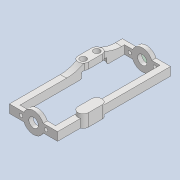
# Autodesk Inventor part: cable_holder_1
Saved by Autodesk Inventor 2020 (Build 240168000, 168)
## iProperties
Created: 2021-07-19
Part Number: cable_holder_1
Material: Generic
Document SubType Name: Modeling
Designer: Shuang Peng
Density: 1 g/cm^3
Appearance: Default
Author: Shuang Peng
Autodesk Inventor part; units mm, degrees
ref_plane "YZ Plane" through (0, 0, 0) normal (1, 0, 0) x (0, 1, 0)
ref_plane "XZ Plane" through (0, 0, 0) normal (0, 1, 0) x (-1, 0, 0)
ref_plane "XY Plane" through (0, 0, 0) normal (0, 0, 1) x (1, 0, 0)
sketch "Sketch1" plane through (0, 0, 0) normal (0, 0, 1) x (1, 0, 0)
  circle A0 centre (0, 0) radius 5
  line L0 (-15, 2) -> (-15, -2)
  line L1 (-15, -2) -> (15, -2)
  line L2 (15, -2) -> (15, 2)
  line L3 (15, 2) -> (-15, 2)
  line L4 (-15, 2) -> (15, -2) construction
  line L5 (-15, -2) -> (15, 2) construction
  point P0 (4.5826, 2)
  point P1 (-4.5826, 2)
  point P2 (-4.5826, -2)
  point P3 (4.5826, -2)
  dimension "d0" = 10
  dimension "d1" = 4
  dimension "d2" = 30
  constraints: 12 end point, 2 midpoint, 2 parallel, 1 centre point, 1 coincident, 1 perpendicular, 1 vertical
  measures "d0" diameter of A0
  measures "d1" distance of L0.start L0.end
  measures "d2" distance of L1.end L0.end
extrude "Extrusion1" add sketch "Sketch1" against normal blind 2
ref_plane "Work Plane1" through (0, 0, -54) normal (0, 0, -1) x (1, 0, 0)
sketch "Sketch2" plane through (0, 0, -54) normal (0, 0, -1) x (1, 0, 0)
  circle A0 centre (0, 0) radius 5
  line L0 (15, 2) -> (15, -2)
  line L1 (15, -2) -> (-15, -2)
  line L2 (-15, -2) -> (-15, 2)
  line L3 (-15, 2) -> (15, 2)
  line L4 (15, 2) -> (-15, -2) construction
  line L5 (15, -2) -> (-15, 2) construction
  point P0 (-4.5826, 2)
  point P1 (-4.5826, -2)
  point P2 (4.5826, -2)
  point P3 (4.5826, 2)
  dimension "d5" = 10
  dimension "d6" = 4
  dimension "d7" = 30
  constraints: 12 end point, 2 midpoint, 2 parallel, 1 centre point, 1 coincident, 1 perpendicular, 1 vertical
  measures "d5" diameter of A0
  measures "d6" distance of L0.start L0.end
  measures "d7" distance of L0.end L1.end
extrude "Extrusion2" add sketch "Sketch2" against normal blind 2
sketch "Sketch3" plane through (4.5826, -2, 0) normal (0, -1, 0) x (1, 0, 0)
  line L0 (0, 0) -> (10.4174, 0) projected
  line L1 (0, 0) -> (0, -2) projected
  line L2 (10.4174, -2) -> (0, -2) projected
  line L3 (10.4174, 0) -> (10.4174, -2) projected
  line L4 (10.4174, -54) -> (0, -54) projected
  line L5 (10.4174, -54) -> (10.4174, -52) projected
  line L6 (0, -52) -> (10.4174, -52) projected
  line L7 (0, -54) -> (0, -52) projected
  line L8 (-9.1652, -54) -> (-19.5826, -54) projected
  line L9 (-9.1652, -54) -> (-9.1652, -52) projected
  line L10 (-19.5826, -52) -> (-9.1652, -52) projected
  line L11 (-19.5826, -54) -> (-19.5826, -52) projected
  line L12 (-19.5826, 0) -> (-9.1652, 0) projected
  line L13 (-19.5826, 0) -> (-19.5826, -2) projected
  line L14 (-9.1652, -2) -> (-19.5826, -2) projected
  line L15 (-9.1652, 0) -> (-9.1652, -2) projected
  line L16 (10.4174, 0) -> (10.4174, -2) projected
  line L17 (10.4174, 0) -> (7.4174, 0)
  line L18 (7.4174, 0) -> (7.4174, -54)
  line L19 (7.4174, -54) -> (10.4174, -54)
  line L20 (10.4174, -54) -> (10.4174, 0)
  line L21 (-19.5826, 0) -> (-19.5826, -2) projected
  line L22 (-19.5826, 0) -> (-16.5826, 0)
  line L23 (-16.5826, 0) -> (-16.5826, -54)
  line L24 (-16.5826, -54) -> (-19.5826, -54)
  line L25 (-19.5826, -54) -> (-19.5826, 0)
  point P0 (-4.5826, 0)
  point P1 (-16.5826, 0)
  point P2 (7.4174, -2)
  point P3 (7.4174, -52)
  dimension "d10" = 3
  dimension "d11" = 54
  dimension "d12" = 3
  dimension "d13" = 54
  constraints: 16 end point, 4 parallel, 2 horizontal, 2 perpendicular
  measures "d10" distance of L19.end L18.end
  measures "d11" distance of L18.end L17.end
  measures "d12" distance of L23.end L24.end
  measures "d13" distance of L22.end L23.end
extrude "Extrusion3" add sketch "Sketch3" against normal up to surface (4 mm away) contours L2 L20 L6 L18 | L8 L11 L10 L23 | L10 L25 L14 L23 | L14 L13 L12 L23
sketch "Sketch4" plane through (0, 0, -54) normal (0, 0, -1) x (-1, 0, 0)
  circle A0 centre (0, 0) radius 2.25
  dimension "d16" = 4.5
  constraints: 1 centre point, 1 coincident
  measures "d16" diameter of A0
extrude "Extrusion4" cut sketch "Sketch4" against normal up to surface (54 mm away)
sketch "Sketch5" plane through (0, 0, 0) normal (0, 0, 1) x (1, 0, 0)
  line L0 (0, 0) -> (-6, 0)
  line L1 (0, 0) -> (6, 0)
  dimension "d19" = 6
  dimension "d20" = 6
  constraints: 4 end point, 2 horizontal
  measures "d19" distance of L0.start L0.end
  measures "d20" distance of L0.start L1.end
hole "Hole1" at (6, 0, 0) at (-6, 0, 0) direction (0, 0, -1) diameter 1.6 depth 100
thicken "Thicken1" operation add thickness 3.5 both sides no extend neighbours yes toward (1, 0, 0) faces at (-12, -0.6667, -35.3333)
thicken "Thicken2" operation add thickness 3.5 both sides no extend neighbours yes toward (-1, 0, 0) faces at (12, -0.6667, -18.6667)
thicken "Thicken3" operation add thickness 3.5 both sides no extend neighbours yes toward (-1, 0, 0) faces at (15, -0.6667, -18)
thicken "Thicken4" operation add thickness 3.5 both sides no extend neighbours yes toward (1, 0, 0) faces at (-15, 0.6667, -18)
sketch "Sketch6" plane through (-4.5826, 2, 0) normal (0, 1, 0) x (1, 0, 0)
  line L0 (0, 0) -> (-6.9174, 0) projected
  line L1 (0, 0) -> (0, 2) projected
  line L2 (-3.9174, 2) -> (0, 2) projected
  line L3 (-3.9174, 52) -> (-3.9174, 2) projected
  line L4 (0, 52) -> (-3.9174, 52) projected
  line L5 (0, 54) -> (0, 52) projected
  line L6 (-6.9174, 54) -> (0, 54) projected
  line L7 (-6.9174, 0) -> (-6.9174, 54) projected
  line L8 (-1.4174, 46.5) -> (1.3129, 46.5) projected
  line L9 (-1.4099, 28.5) -> (10.5826, 28.5) projected
  line L10 (-6.9174, 54) -> (0, 54) projected
  line L11 (-6.9174, 54) -> (-6.9174, 46.5)
  line L12 (-6.9174, 0) -> (-6.9174, 54) projected
  line L13 (-6.9174, 46.5) -> (-6.9174, 37.5)
  line L14 (-6.9174, 37.5) -> (-3.9174, 37.5)
  line L15 (-3.9174, 37.5) -> (-3.9174, 40.75)
  line L16 (-3.9174, 52) -> (-3.9174, 2) projected
  line L17 (-3.9174, 37.5) -> (-3.9174, 34.25)
  circle A0 centre (-3.9174, 40.75) radius 3
  circle A1 centre (-3.9174, 34.25) radius 3
  line L18 (-3.9174, 34.25) -> (-5.9174, 34.25)
  line L19 (-5.9174, 34.25) -> (-5.9174, 40.75)
  line L20 (-5.9174, 34.25) -> (-5.9174, 40.75) construction
  line L21 (-2.9174, 34.25) -> (-2.9174, 40.75)
  line L22 (-8.9174, 40.75) -> (-8.9174, 34.25)
  arc A2 (-8.9174, 34.25) -> (-2.9174, 34.25) centre (-5.9174, 34.25) ccw
  arc A3 (-2.9174, 40.75) -> (-8.9174, 40.75) centre (-5.9174, 40.75) ccw
  point P0 (4.5826, 0)
  point P1 (-5.9174, 37.5)
  dimension "d36" = 7.5
  dimension "d37" = 9
  dimension "d38" = 3
  dimension "d39" = 3.25
  dimension "d40" = 3.25
  dimension "d41" = 6
  dimension "d42" = 6
  dimension "d43" = 2
  dimension "d44" = 6.5
  dimension "d45" = 6
  constraints: 22 end point, 5 point on line, 4 centre point, 4 point on circle, 4 tangent, 2 coincident, 2 equal length, 1 horizontal, 1 midpoint, 1 vertical
  measures "d36" distance of L6.start L11.end
  measures "d37" distance of L11.end L13.end
  measures "d38" distance of L13.end L14.end
  measures "d39" distance of L14.end L15.end
  measures "d40" distance of L14.end L17.end
  measures "d41" diameter of A0
  measures "d42" diameter of A1
  measures "d43" distance of L18.start L18.end
  measures "d44" distance of L18.end L19.end
  measures "d45" diameter of A3
extrude "Extrusion5" add sketch "Sketch6" against normal up to surface (4 mm away) contours A2 L22 A3 L7 | L7 A1 A2 | L7 L14 L19 A1 | A1 L19 L18 L3 A2 | L7 A0 L19 L14 | L19 L14 L3 A1 | A1 L3 L18 L19 | L3 A1 L21 A2 | L7 A3 A0 | A0 A3 L3 | L19 A0 L3 L14 | L3 A0 L21 A1 | A0 L3 A3 L21 picked at (-3.2507, 35.1928) picked at (-4.6568, 42.1686) picked at (-3.2507, 39.8072)
sketch "Sketch7" plane through (4.5826, 2, 0) normal (0, 1, 0) x (1, 0, 0)
  line L0 (6.9174, 0) -> (0, 0) projected
  line L1 (6.9174, 0) -> (6.9174, 54) projected
  line L2 (0, 54) -> (6.9174, 54) projected
  line L3 (0, 54) -> (0, 52) projected
  line L4 (3.9174, 52) -> (0, 52) projected
  line L5 (3.9174, 2) -> (3.9174, 52) projected
  line L6 (0, 2) -> (3.9174, 2) projected
  line L7 (0, 0) -> (0, 2) projected
  line L8 (0.625, 7.5) -> (-7.1532, 7.5) projected
  line L9 (6.9174, 0) -> (6.9174, 54) projected
  line L10 (6.9174, 0) -> (6.9174, 7.5)
  line L11 (6.9174, 7.5) -> (6.9174, 16.5)
  line L12 (6.9174, 16.5) -> (3.9174, 16.5)
  line L13 (3.9174, 2) -> (3.9174, 52) projected
  line L14 (3.9174, 16.5) -> (5.9174, 16.5)
  line L15 (5.9174, 16.5) -> (5.9174, 13.25)
  line L16 (5.9174, 13.25) -> (5.9174, 19.75) construction
  line L17 (8.9174, 13.25) -> (8.9174, 19.75)
  line L18 (2.9174, 19.75) -> (2.9174, 13.25)
  arc A0 (2.9174, 13.25) -> (8.9174, 13.25) centre (5.9174, 13.25) ccw
  arc A1 (8.9174, 19.75) -> (2.9174, 19.75) centre (5.9174, 19.75) ccw
  point P0 (-4.5826, 0)
  point P1 (5.9174, 16.5)
  point P2 (6.9174, 22.5784)
  point P3 (6.9174, 10.4216)
  point P4 (3.9174, 11.0139)
  point P5 (3.9174, 21.9861)
  dimension "d48" = 7.5
  dimension "d49" = 9
  dimension "d50" = 2
  dimension "d51" = 3.25
  dimension "d52" = 6.5
  dimension "d53" = 6
  constraints: 18 end point, 4 point on circle, 4 tangent, 3 point on line, 2 centre point, 2 perpendicular, 1 collinear, 1 midpoint, 1 parallel, 1 vertical
  measures "d48" distance of L0.start L10.end
  measures "d49" distance of L10.end L11.end
  measures "d50" distance of L12.end L14.end
  measures "d51" distance of L14.end L15.end
  measures "d52" distance of L15.end L16.end
  measures "d53" diameter of A1
extrude "Extrusion6" add sketch "Sketch7" against normal up to surface (4 mm away) contours L1 A1 L17 A0 | A0 L18 A1 L5
sketch "Sketch9" plane through (-4.5826, -2, -2) normal (0, -1, 0) x (1, 0, 0)
  line L0 (-3.9174, -30.0139) -> (-3.9174, 0) projected
  line L1 (0, 0) -> (-3.9174, 0) projected
  line L2 (0, 2) -> (0, 0) projected
  line L3 (-6.9174, 2) -> (0, 2) projected
  line L4 (-6.9174, 2) -> (-6.9174, -29.4216) projected
  arc A0 (-6.9174, -29.4216) -> (-8.9174, -32.25) centre (-5.9174, -32.25) ccw projected
  line L5 (-8.9174, -38.75) -> (-8.9174, -32.25) projected
  arc A1 (-8.9174, -38.75) -> (-6.9174, -41.5784) centre (-5.9174, -38.75) ccw projected
  line L6 (-6.9174, -41.5784) -> (-6.9174, -52) projected
  line L7 (0, -52) -> (-6.9174, -52) projected
  line L8 (0, -52) -> (0, -50) projected
  line L9 (-3.9174, -50) -> (0, -50) projected
  line L10 (-3.9174, -50) -> (-3.9174, -40.9861) projected
  arc A2 (-3.9174, -40.9861) -> (-2.9174, -38.75) centre (-5.9174, -38.75) ccw projected
  line L11 (-2.9174, -32.25) -> (-2.9174, -38.75) projected
  arc A3 (-2.9174, -32.25) -> (-3.9174, -30.0139) centre (-5.9174, -32.25) ccw projected
  line L12 (-5.9174, -38.75) -> (-5.9174, -32.25) construction
  line L13 (-2.4174, -38.75) -> (-2.4174, -32.25)
  line L14 (-9.4174, -32.25) -> (-9.4174, -38.75)
  arc A4 (-9.4174, -38.75) -> (-2.4174, -38.75) centre (-5.9174, -38.75) ccw
  arc A5 (-2.4174, -32.25) -> (-9.4174, -32.25) centre (-5.9174, -32.25) ccw
  point P0 (4.5826, 2)
  point P1 (-5.9174, -35.5)
  dimension "d60" = 7
  constraints: 8 end point, 4 point on circle, 4 tangent, 2 centre point, 1 midpoint, 1 parallel, 1 vertical
  measures "d60" diameter of A5
extrude "Extrusion8" cut sketch "Sketch9" against normal blind 3 contours A3 L11 A2 L10 A4 L6 A1 L5 A0 L4 A5 L0 | L0 A5 L13 A4 L10 A2 L11 A3 | L4 A0 L5 A1 L6 A4 L14 A5
sketch "Sketch10" plane through (-4.5826, 1, -2) normal (0, -1, 0) x (1, 0, 0)
  arc A0 (-6.9174, -29.4216) -> (-8.9174, -32.25) centre (-5.9174, -32.25) ccw projected
  line L0 (-8.9174, -38.75) -> (-8.9174, -32.25) projected
  arc A1 (-8.9174, -38.75) -> (-6.9174, -41.5784) centre (-5.9174, -38.75) ccw projected
  arc A2 (-3.9174, -40.9861) -> (-2.9174, -38.75) centre (-5.9174, -38.75) ccw projected
  line L1 (-2.9174, -32.25) -> (-2.9174, -38.75) projected
  arc A3 (-2.9174, -32.25) -> (-3.9174, -30.0139) centre (-5.9174, -32.25) ccw projected
  circle A4 centre (-5.9174, -38.75) radius 1.5
  circle A5 centre (-5.9174, -32.25) radius 1.5
  line L2 (-6.9174, -29.4216) -> (-6.9174, -28.8959) projected
  line L3 (-6.9174, -42.1041) -> (-6.9174, -41.5784) projected
  arc A6 (-6.9174, -42.1041) -> (-3.9174, -41.6223) centre (-5.9174, -38.75) ccw projected
  line L4 (-3.9174, -40.9861) -> (-3.9174, -41.6223) projected
  line L5 (-3.9174, -29.3777) -> (-3.9174, -30.0139) projected
  arc A7 (-3.9174, -29.3777) -> (-6.9174, -28.8959) centre (-5.9174, -32.25) ccw projected
  point P0 (4.5826, 2)
  dimension "d66" = 3
  dimension "d67" = 3
  constraints: 2 centre point, 2 coincident
  measures "d66" diameter of A4
  measures "d67" diameter of A5
extrude "Extrusion9" cut sketch "Sketch10" against normal blind 3 contours A4 | A5
sketch "Sketch11" plane through (-4.5826, -2, -54) normal (0, -1, 0) x (1, 0, 0)
  arc A0 (-6.9174, 9.8959) -> (-3.9174, 10.3777) centre (-5.9174, 13.25) ccw projected
  line L0 (-6.9174, 9.8959) -> (-6.9174, 0) projected
  line L1 (0, 0) -> (-6.9174, 0) projected
  line L2 (0, 0) -> (0, 2) projected
  line L3 (-3.9174, 2) -> (0, 2) projected
  line L4 (-3.9174, 2) -> (-3.9174, 10.3777) projected
  arc A1 (-3.9174, 22.6223) -> (-6.9174, 23.1041) centre (-5.9174, 19.75) ccw projected
  line L5 (-3.9174, 22.6223) -> (-3.9174, 52) projected
  line L6 (0, 52) -> (-3.9174, 52) projected
  line L7 (0, 54) -> (0, 52) projected
  line L8 (-6.9174, 54) -> (0, 54) projected
  line L9 (-6.9174, 54) -> (-6.9174, 23.1041) projected
  line L10 (-5.9174, 13.25) -> (-5.9174, 19.75) construction
  line L11 (-2.4174, 13.25) -> (-2.4174, 19.75)
  line L12 (-9.4174, 19.75) -> (-9.4174, 13.25)
  arc A2 (-9.4174, 13.25) -> (-2.4174, 13.25) centre (-5.9174, 13.25) ccw
  arc A3 (-2.4174, 19.75) -> (-9.4174, 19.75) centre (-5.9174, 19.75) ccw
  line L13 (-5.9174, 13.25) -> (-5.9174, 19.75) construction
  line L14 (-1.4174, 13.25) -> (-1.4174, 19.75)
  line L15 (-10.4174, 19.75) -> (-10.4174, 13.25)
  arc A4 (-10.4174, 13.25) -> (-1.4174, 13.25) centre (-5.9174, 13.25) ccw
  arc A5 (-1.4174, 19.75) -> (-10.4174, 19.75) centre (-5.9174, 19.75) ccw
  point P0 (4.5826, 54)
  point P1 (-5.9174, 16.5)
  point P2 (-5.9174, 16.5)
  point P3 (-3.9174, 10.3777)
  point P4 (-3.9174, 9.2189)
  point P5 (-3.9174, 23.7811)
  point P6 (-3.9174, 22.6223)
  dimension "d70" = 7
  dimension "d71" = 9
  constraints: 16 end point, 8 point on circle, 8 tangent, 4 centre point, 2 midpoint, 2 parallel, 2 vertical, 1 concentric
  measures "d70" diameter of A3
  measures "d71" diameter of A5
extrude "Extrusion10" add sketch "Sketch11" against normal up to surface (4 mm away) contours A2 L11 A3 L5 A5 L14 A4 L4
thicken "Thicken5" operation add thickness 0.5 both sides no extend neighbours yes toward (0.8468765, 0, -0.5317897) faces at (-7.9594, 1.3333, -42.3454)
sketch "Sketch12" plane through (4.5826, -2, -2) normal (0, -1, 0) x (1, 0, 0)
  line L0 (0, 2) -> (6.9174, 2) projected
  line L1 (0, 2) -> (0, 0) projected
  line L2 (3.9174, 0) -> (0, 0) projected
  line L3 (3.9174, 0) -> (3.9174, -9.0139) projected
  arc A0 (3.9174, -9.0139) -> (2.9174, -11.25) centre (5.9174, -11.25) ccw projected
  line L4 (2.9174, -17.75) -> (2.9174, -11.25) projected
  arc A1 (2.9174, -17.75) -> (3.9174, -19.9861) centre (5.9174, -17.75) ccw projected
  line L5 (3.9174, -19.9861) -> (3.9174, -50) projected
  line L6 (0, -50) -> (3.9174, -50) projected
  line L7 (0, -52) -> (0, -50) projected
  line L8 (6.9174, -52) -> (0, -52) projected
  line L9 (6.9174, -20.5784) -> (6.9174, -52) projected
  arc A2 (6.9174, -20.5784) -> (8.9174, -17.75) centre (5.9174, -17.75) ccw projected
  line L10 (8.9174, -11.25) -> (8.9174, -17.75) projected
  arc A3 (8.9174, -11.25) -> (6.9174, -8.4216) centre (5.9174, -11.25) ccw projected
  line L11 (6.9174, 2) -> (6.9174, -8.4216) projected
  line L12 (5.9174, -17.75) -> (5.9174, -11.25) construction
  line L13 (9.4174, -17.75) -> (9.4174, -11.25)
  line L14 (2.4174, -11.25) -> (2.4174, -17.75)
  arc A4 (2.4174, -17.75) -> (9.4174, -17.75) centre (5.9174, -17.75) ccw
  arc A5 (9.4174, -11.25) -> (2.4174, -11.25) centre (5.9174, -11.25) ccw
  point P0 (-4.5826, 2)
  point P1 (5.9174, -14.5)
  dimension "d76" = 6.5
  dimension "d77" = 7
  constraints: 8 end point, 4 point on circle, 4 tangent, 2 centre point, 1 midpoint, 1 parallel, 1 vertical
  measures "d76" distance of L12.start L12.end
  measures "d77" diameter of A5
extrude "Extrusion11" cut sketch "Sketch12" against normal blind 3 contours A5 L13 A4 L9 A2 L10 A3 L11 | L11 A3 L10 A2 L9 A4 L5 A1 L4 A0 L3 A5 | L3 A0 L4 A1 L5 A4 L14 A5
sketch "Sketch13" plane through (4.5826, 1, -2) normal (0, -1, 0) x (1, 0, 0)
  line L0 (3.9174, -9.0139) -> (3.9174, -8.3777) projected
  arc A0 (3.9174, -9.0139) -> (2.9174, -11.25) centre (5.9174, -11.25) ccw projected
  line L1 (2.9174, -17.75) -> (2.9174, -11.25) projected
  arc A1 (2.9174, -17.75) -> (3.9174, -19.9861) centre (5.9174, -17.75) ccw projected
  line L2 (3.9174, -20.6223) -> (3.9174, -19.9861) projected
  arc A2 (3.9174, -20.6223) -> (6.9174, -21.1041) centre (5.9174, -17.75) ccw projected
  line L3 (6.9174, -20.5784) -> (6.9174, -21.1041) projected
  arc A3 (6.9174, -20.5784) -> (8.9174, -17.75) centre (5.9174, -17.75) ccw projected
  line L4 (8.9174, -11.25) -> (8.9174, -17.75) projected
  arc A4 (8.9174, -11.25) -> (6.9174, -8.4216) centre (5.9174, -11.25) ccw projected
  line L5 (6.9174, -7.8959) -> (6.9174, -8.4216) projected
  arc A5 (6.9174, -7.8959) -> (3.9174, -8.3777) centre (5.9174, -11.25) ccw projected
  point P0 (-4.5826, 2)
hole "Hole2" at (10.5, 1, -19.75) at (10.5, 1, -13.25) direction (0, 1, 0) diameter 3 depth 100
sketch "Sketch14" plane through (4.5826, -2, -54) normal (0, -1, 0) x (1, 0, 0)
  arc A0 (3.9174, 31.3777) -> (6.9174, 30.8959) centre (5.9174, 34.25) ccw projected
  line L0 (3.9174, 31.3777) -> (3.9174, 2) projected
  line L1 (0, 2) -> (3.9174, 2) projected
  line L2 (0, 0) -> (0, 2) projected
  line L3 (6.9174, 0) -> (0, 0) projected
  line L4 (6.9174, 30.8959) -> (6.9174, 0) projected
  arc A1 (6.9174, 44.1041) -> (3.9174, 43.6223) centre (5.9174, 40.75) ccw projected
  line L5 (6.9174, 54) -> (6.9174, 44.1041) projected
  line L6 (0, 54) -> (6.9174, 54) projected
  line L7 (0, 54) -> (0, 52) projected
  line L8 (3.9174, 52) -> (0, 52) projected
  line L9 (3.9174, 52) -> (3.9174, 43.6223) projected
  circle A2 centre (5.9174, 40.75) radius 1.5 projected
  line L10 (5.9174, 34.25) -> (5.9174, 40.75) construction
  line L11 (9.4174, 34.25) -> (9.4174, 40.75)
  line L12 (2.4174, 40.75) -> (2.4174, 34.25)
  arc A3 (2.4174, 34.25) -> (9.4174, 34.25) centre (5.9174, 34.25) ccw
  arc A4 (9.4174, 40.75) -> (2.4174, 40.75) centre (5.9174, 40.75) ccw
  line L13 (5.9174, 34.25) -> (5.9174, 40.75) construction
  line L14 (10.9174, 34.25) -> (10.9174, 40.75)
  line L15 (0.9174, 40.75) -> (0.9174, 34.25)
  arc A5 (0.9174, 34.25) -> (10.9174, 34.25) centre (5.9174, 34.25) ccw
  arc A6 (10.9174, 40.75) -> (0.9174, 40.75) centre (5.9174, 40.75) ccw
  point P0 (-4.5826, 54)
  point P1 (5.9174, 37.5)
  point P2 (5.9174, 37.5)
  point P3 (3.9174, 29.6674)
  point P4 (3.9174, 31.3777)
  point P5 (3.9174, 43.6223)
  point P6 (3.9174, 45.3326)
  dimension "d87" = 7
  dimension "d88" = 1.5
  constraints: 16 end point, 8 point on circle, 8 tangent, 4 centre point, 3 equal length, 2 midpoint, 1 vertical
  measures "d87" diameter of A4
  measures "d88" radial gap between concentric circles of A6 A4
extrude "Extrusion12" add sketch "Sketch14" against normal up to surface (4 mm away) contours L0 A5 L15 A6 L9 A4 L12 A3
thicken "Thicken6" operation add thickness 0.5 both sides no extend neighbours yes toward (-0.9609569, 0, -0.276698) faces at (7.6171, 1.3333, -20.5801)
thicken "Thicken7" operation add thickness 0.5 both sides no extend neighbours yes toward (0.8297542, 0, -0.558129) faces at (-6.7661, -0.6667, -43.2616)
body "Solid1"
